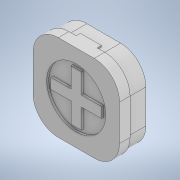
# Autodesk Inventor part: Health-Item-Pack
Saved by Autodesk Inventor 2020 (Build 240168000, 168)
## iProperties
Created: 2019-09-14
Part Number: Health-Item-Pack
Material: Generic
Document SubType Name: Modeling
Designer: Victor
Density: 1 g/cm^3
Appearance: Default
Author: Victor
Autodesk Inventor part; units mm, degrees
ref_plane "YZ Plane" through (0, 0, 0) normal (1, 0, 0) x (0, 1, 0)
ref_plane "XZ Plane" through (0, 0, 0) normal (0, 1, 0) x (-1, 0, 0)
ref_plane "XY Plane" through (0, 0, 0) normal (0, 0, 1) x (1, 0, 0)
sketch "Sketch1" plane through (0, 0, 0) normal (0, 0, 1) x (1, 0, 0)
  line L0 (-10, -10) -> (10, -10)
  line L1 (10, -10) -> (10, 10)
  line L2 (10, 10) -> (-10, 10)
  line L3 (-10, 10) -> (-10, -10)
  line L4 (-10, -10) -> (10, 10) construction
  line L5 (10, -10) -> (-10, 10) construction
  point P0 (0, 0)
  dimension "d0" = 20
  dimension "d1" = 20
  constraints: 12 end point, 2 midpoint, 2 parallel, 1 horizontal, 1 perpendicular
  measures "d0" distance of L1.end L2.end
  measures "d1" distance of L0.end L1.end
extrude "Extrusion1" add sketch "Sketch1" along normal blind 4
sketch "Sketch2" plane through (0, 0, 4) normal (0, 0, 1) x (1, 0, 0)
  line L0 (-10.25, 10.25) -> (10.25, 10.25)
  line L1 (10.25, 10.25) -> (10.25, -10.25)
  line L2 (10.25, -10.25) -> (-10.25, -10.25)
  line L3 (-10.25, -10.25) -> (-10.25, 10.25)
  line L4 (-10.25, 10.25) -> (10.25, -10.25) construction
  line L5 (10.25, 10.25) -> (-10.25, -10.25) construction
  point P0 (0, 0)
  dimension "d4" = 20.5
  dimension "d5" = 20.5
  constraints: 12 end point, 2 midpoint, 2 parallel, 1 horizontal, 1 perpendicular
  measures "d4" distance of L1.end L2.end
  measures "d5" distance of L0.end L1.end
extrude "Extrusion2" add sketch "Sketch2" along normal blind 2.5
fillet "Fillet1" radius 6 8 edges at (-10, 10, 2) (10, 10, 2) (-10, -10, 2) (-10.25, -10.25, 5.25) (-10.25, 10.25, 5.25) (10.25, 10.25, 5.25) (10, -10, 2) (10.25, -10.25, 5.25)
sketch "Sketch3" plane through (0, 0, 4) normal (0, 0, -1) x (-1, 0, 0)
  line L0 (-4.25, 10.25) -> (4.25, 10.25) projected
  line L1 (2.5, 9.75) -> (-2.5, 9.75)
  line L2 (-2.5, 9.75) -> (-2.5, 10.25)
  line L3 (-2.5, 10.25) -> (2.5, 10.25)
  line L4 (2.5, 10.25) -> (2.5, 9.75)
  line L5 (-4, 10) -> (4, 10) projected
  line L6 (2.5, 9.75) -> (-2.5, 10.25) construction
  line L7 (-2.5, 9.75) -> (2.5, 10.25) construction
  point P0 (0, 0)
  point P1 (0, 10)
  dimension "d9" = 5
  constraints: 12 end point, 3 midpoint, 2 parallel, 1 horizontal, 1 perpendicular, 1 point on line
  measures "d9" distance of L2.end L3.end
extrude "Extrusion3" add sketch "Sketch3" along normal blind 1
sketch "Sketch4" plane through (0, 0, 6.5) normal (0, 0, 1) x (1, 0, 0)
  circle A0 centre (0, 0) radius 7
  line L0 (-6, -1.25) -> (6, -1.25)
  line L1 (6, -1.25) -> (6, 1.25)
  line L2 (6, 1.25) -> (-6, 1.25)
  line L3 (-6, 1.25) -> (-6, -1.25)
  line L4 (-6, -1.25) -> (6, 1.25) construction
  line L5 (6, -1.25) -> (-6, 1.25) construction
  line L6 (1.25, -6) -> (-1.25, -6)
  line L7 (-1.25, -6) -> (-1.25, 6)
  line L8 (-1.25, 6) -> (1.25, 6)
  line L9 (1.25, 6) -> (1.25, -6)
  line L10 (1.25, -6) -> (-1.25, 6) construction
  line L11 (-1.25, -6) -> (1.25, 6) construction
  point P0 (-1.25, 1.25)
  point P1 (1.25, 1.25)
  point P2 (1.25, -1.25)
  point P3 (-1.25, -1.25)
  dimension "d12" = 14
  dimension "d13" = 12
  dimension "d14" = 2.5
  dimension "d15" = 2.5
  dimension "d16" = 12
  constraints: 24 end point, 4 midpoint, 4 parallel, 2 horizontal, 2 perpendicular, 1 centre point, 1 coincident
  measures "d12" diameter of A0
  measures "d13" distance of L2.end L1.end
  measures "d14" distance of L1.end L0.end
  measures "d15" distance of L7.end L8.end
  measures "d16" distance of L6.end L7.end
extrude "Extrusion4" cut sketch "Sketch4" against normal blind 0.5
equation "\"d1\" = d0"
equation "\"d5\" = d4"
body "Solid1"
